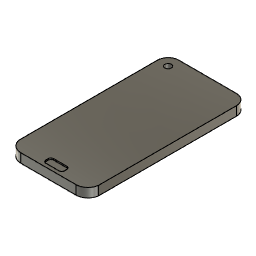
iPhone (Autodesk Fusion 360 design; units mm, degrees)
Autodesk Fusion 360 part; units mm, degrees
sketch "phone" plane through (0, 0, 0) normal (0, 0, 1) x (1, 0, 0)
  line L0 (-42, -60) -> (-21, -60)
  arc A0 (-21, -60) -> (-12, -52) centre (-21, -50.9375) ccw
  line L1 (-12, -52) -> (-12, 53)
  arc A1 (-12, 53) -> (-20, 61) centre (-20, 53) ccw
  line L2 (-20, 61) -> (-42, 61)
  line L3 (-64, 61) -> (-42, 61)
  arc A2 (-64, 61) -> (-72, 53) centre (-64, 53) ccw
  line L4 (-72, -52) -> (-72, 53)
  arc A3 (-72, -52) -> (-63, -60) centre (-63, -50.9375) ccw
  line L5 (-42, -60) -> (-63, -60)
  constraint horizontal L0
  constraint tangent L0 A0
  constraint perpendicular L0 L1
  constraint tangent L1 A1
  constraint tangent A1 L2
  constraint perpendicular L1 L2
extrude "Extrude1" add sketch "phone" along normal blind 6.91
hole "Hole1" at (-64, 53, 6.91) direction (0, 0, -1) diameter 5 depth 40 tip angle 118
sketch "button" plane through (0, 0, 6.91) normal (0, 0, 1) x (-1, 0, 0)
  circle A0 centre (64, -53) radius 2.5
  arc A1 (21, 60) -> (12, 52) centre (21, 50.9375) ccw
  line L0 (12, 52) -> (12, -53)
  arc A2 (12, -53) -> (20, -61) centre (20, -53) ccw
  line L1 (20, -61) -> (64, -61)
  arc A3 (64, -61) -> (72, -53) centre (64, -53) ccw
  line L2 (72, -53) -> (72, 52)
  arc A4 (72, 52) -> (63, 60) centre (63, 50.9375) ccw
  line L3 (63, 60) -> (21, 60)
  line L4 (46.6846, 51.3855) -> (36.5241, 51.3855)
  line L5 (34.5241, 53.3855) -> (34.5241, 55.3855)
  line L6 (36.5241, 57.3855) -> (46.6846, 57.3855)
  line L7 (48.6846, 55.3855) -> (48.6846, 53.3855)
  arc A5 (46.6846, 51.3855) -> (48.6846, 53.3855) centre (46.6846, 53.3855) ccw
  arc A6 (48.6846, 55.3855) -> (46.6846, 57.3855) centre (46.6846, 55.3855) ccw
  arc A7 (34.5241, 53.3855) -> (36.5241, 51.3855) centre (36.5241, 53.3855) ccw
  arc A8 (36.5241, 57.3855) -> (34.5241, 55.3855) centre (36.5241, 55.3855) ccw
  dimension "d6" = 2
  constraint horizontal L4
  constraint vertical L5
  constraint horizontal L6
  constraint vertical L7
  constraint tangent L4 A5
  constraint tangent L7 A5
  constraint tangent L6 A6
  constraint tangent L7 A6
  constraint equal A5 A6
  constraint tangent L4 A7
  constraint tangent L5 A7
  constraint equal A5 A7
  constraint tangent L5 A8
  constraint tangent L6 A8
  constraint equal A5 A8
  measures "d6" radius of A5
extrude "Extrude2" cut sketch "button" against normal blind 1 contours L4 L5 L6 L7 A5 A6 A7 A8
named bodies: "phone"
